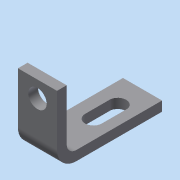
# Autodesk Inventor part: dsub37Bracket
Saved by Autodesk Inventor 2016 (Build 200138000, 138)
## iProperties
Created: 2016-10-03
Part Number: dsub37Bracket
Material: Generic
Document SubType Name: Sheet Metal
Designer: Zara
Density: 1 g/cm^3
Sheet Metal Rule: Default
Appearance: Default
Author: Zara
Autodesk Inventor part; units mm, degrees
ref_plane "YZ Plane" through (0, 0, 0) normal (1, 0, 0) x (0, 1, 0)
ref_plane "XZ Plane" through (0, 0, 0) normal (0, 1, 0) x (-1, 0, 0)
ref_plane "XY Plane" through (0, 0, 0) normal (0, 0, 1) x (1, 0, 0)
sketch "Sketch1" plane through (0, 0, 0) normal (0, 1, 0) x (-1, 0, 0)
  line L0 (-3.0226, 8.128) -> (3.0226, 8.128)
  line L1 (3.0226, 8.128) -> (3.0226, -8.128)
  line L2 (3.0226, -8.128) -> (-3.0226, -8.128)
  line L3 (-3.0226, -8.128) -> (-3.0226, 8.128)
  line L4 (-3.0226, 8.128) -> (3.0226, -8.128) construction
  line L5 (3.0226, 8.128) -> (-3.0226, -8.128) construction
  line L6 (1.1394, -0.381) -> (1.1394, -4.3425)
  line L7 (-1.4442, -0.381) -> (-1.4442, -4.3425)
  arc A0 (-1.4442, -4.3425) -> (1.1394, -4.3425) centre (-0.1524, -4.1402) ccw
  arc A1 (1.1394, -0.381) -> (-1.4442, -0.381) centre (-0.1524, -0.381) ccw
  line L8 (0, 9.1418) -> (0, -10.0518)
  point P0 (0, 0)
  dimension "d0" = 16.256
  dimension "d1" = 6.0452
  dimension "d2" = 3.9878
  dimension "d3" = 7.747
  dimension "d4" = 3.175
  dimension "d5" = 3.175
  measures "d0" distance of L0.end L1.end
  measures "d1" distance of L1.end L2.end
  measures "d2" distance from line of A0.centre L2
  measures "d3" distance from line of A1.centre L2
  measures "d4" distance from line of A0.centre L1
  measures "d5" distance from line of L1 A1.centre
extrude "Plate1" add sketch "Sketch1" along normal blind 1.4986 contours L0 L8 A1 L7 A0 L2 L3 | L0 L1 L2 L8 A0 L6 A1
sketch "Sketch2" plane through (3.0226, 0, 6.6294) normal (0, 0, 1) x (1, 0, 0)
  line L0 (-6.0452, 0) -> (0, 0)
  line L1 (0, 0) -> (0, 10.922)
  line L2 (0, 10.922) -> (-6.0452, 10.922)
  line L3 (-6.0452, 10.922) -> (-6.0452, 0)
  constraints: 6 end point, 1 horizontal, 1 perpendicular, 1 vertical
edge flange "Flange1" height 10.922 angle 90 thickness 1.4986 bend radius 1.4986 thickness toward (0, 0, 1) relief tear relief width 1.4986 relief depth 0.7493 edges at (0, 1.4986, 8.128) wall of the first edge with corners at (-3.0226, 0, 6.6294) (3.0226, 0, 6.6294) (3.0226, 10.922, 6.6294) (-3.0226, 10.922, 6.6294)
bend "Bend1"
corner "Corner1"
sketch "Sketch4" plane through (3.0226, 10.922, 6.6294) normal (0, 0, -1) x (-1, 0, 0)
  circle A0 centre (3.0226, -2.54) radius 1.4224
  line L0 (6.0452, 0) -> (0, 0) projected
  point P0 (3.0226, -10.922)
  dimension "d21" = 2.54
  dimension "d22" = 2.8448
  constraints: 1 centre point
  measures "d21" distance from line of L0 A0.centre
  measures "d22" diameter of A0
extrude "Extrusion3" cut sketch "Sketch4" against normal blind 1.4986
equation "\"d11\" = BendReliefWidth"
equation "\"d12\" = BendReliefDepth"
equation "\"d13\" = MinimumRemnant"
equation "\"d14\" = BendRadius"
equation "\"d17\" = BendRadius"
equation "\"d18\" = CornerReliefSize"
equation "\"d19\" = GapSize"
equation "\"d20\" = JacobiRadiusSize"
equation "\"BendRadius\" = Thickness"
equation "\"BendReliefWidth\" = Thickness"
equation "\"BendReliefDepth\" = 0.5 * Thickness"
equation "\"CornerReliefSize\" = 4 * Thickness"
equation "\"MinimumRemnant\" = 2 * Thickness"
equation "\"TransitionRadius\" = BendRadius"
equation "\"JacobiRadiusSize\" = Thickness"
equation "\"GapSize\" = Thickness"
equation "\"d10\" = BendRadius"
equation "\"Thickness\" = 1.4986"
body "Solid3"
